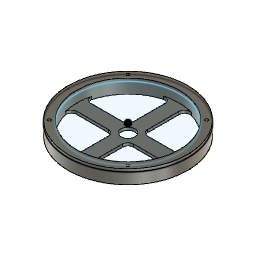
main_body_43mm_diameter v2 (Autodesk Fusion 360 design; units mm, degrees)
Autodesk Fusion 360 part; units mm, degrees
sketch "Sketch1" plane through (0, 0, 0) normal (0, 0, 1) x (1, 0, 0)
  circle A0 centre (0, 0) radius 21.5
  circle A1 centre (0, 0) radius 18.5
  circle A2 centre (0, 0) radius 2.5
  line L0 (-2.5, 4.5) -> (-2.5, 15.8622)
  line L1 (2.5, 15.8622) -> (2.5, 4.5)
  line L2 (4.5, -2.5) -> (15.8806, -2.5)
  line L3 (15.8806, 2.5) -> (4.5, 2.5)
  line L4 (-2.5, -4.5) -> (-2.5, -15.8473)
  line L5 (2.5, -15.8473) -> (2.5, -4.5)
  line L6 (-4.5, -2.5) -> (-15.892, -2.5)
  line L7 (-15.9057, 2.5) -> (-4.5, 2.5)
  arc A3 (2.5, 4.5) -> (4.5, 2.5) centre (4.5, 4.5) ccw
  arc A4 (4.5, -2.5) -> (2.5, -4.5) centre (4.5, -4.5) ccw
  arc A5 (-2.5, -4.5) -> (-4.5, -2.5) centre (-4.5, -4.5) ccw
  arc A6 (-4.5, 2.5) -> (-2.5, 4.5) centre (-4.5, 4.5) ccw
  line L8 (-17.8692, 4.8804) -> (-17.9378, 4.526)
  line L9 (-17.8533, -4.8912) -> (-17.8867, -4.7239)
  arc A7 (-17.8692, 4.8804) -> (-15.9057, 2.5) centre (-15.9057, 4.5) ccw
  arc A8 (-15.892, -2.5) -> (-17.8533, -4.8912) centre (-15.892, -4.5) ccw
  line L10 (-4.926, -17.8014) -> (-5.3564, -17.7076)
  line L11 (4.926, -17.8014) -> (5.3564, -17.7076)
  arc A9 (-4.926, -17.8014) -> (-2.5, -15.8473) centre (-4.5, -15.8473) ccw
  arc A10 (2.5, -15.8473) -> (4.926, -17.8014) centre (4.5, -15.8473) ccw
  line L12 (17.8401, -4.9002) -> (17.8428, -4.8872)
  line L13 (17.8401, 4.9002) -> (17.8428, 4.8872)
  arc A11 (15.8806, 2.5) -> (17.8401, 4.9002) centre (15.8806, 4.5) ccw
  arc A12 (17.8401, -4.9002) -> (15.8806, -2.5) centre (15.8806, -4.5) ccw
  line L14 (4.9145, 17.8188) -> (5.1482, 17.7693)
  line L15 (-4.9145, 17.8188) -> (-5.1482, 17.7693)
  arc A13 (-2.5, 15.8622) -> (-4.9145, 17.8188) centre (-4.5, 15.8622) ccw
  arc A14 (4.9145, 17.8188) -> (2.5, 15.8622) centre (4.5, 15.8622) ccw
  dimension "d1" = 43
  dimension "d2" = 37
  dimension "d3" = 5
  dimension "d6" = 2
  dimension "d7" = 2
  dimension "d8" = 2
  dimension "d9" = 2
  dimension "d10" = 2
  dimension "d11" = 2
  dimension "d12" = 2
  dimension "d13" = 2
  dimension "d14" = 2
  dimension "d15" = 2
  dimension "d16" = 2
  dimension "d17" = 2
  constraint concentric A0 A1
  constraint concentric A1 A2
  constraint vertical L0
  constraint vertical L1
  constraint horizontal L2
  constraint horizontal L3
  constraint vertical L4
  constraint vertical L5
  constraint horizontal L6
  constraint horizontal L7
  constraint tangent L1 A3
  constraint tangent L3 A3
  constraint tangent L2 A4
  constraint tangent L5 A4
  constraint tangent L6 A5
  constraint tangent L4 A5
  constraint tangent L7 A6
  constraint tangent L0 A6
  constraint coincident A1 L8.end
  constraint coincident A1 L9.end
  constraint tangent L8 A7
  constraint tangent L7 A7
  constraint tangent L9 A8
  constraint tangent L6 A8
  constraint coincident A1 L10.end
  constraint coincident A1 L11.end
  constraint tangent L10 A9
  constraint tangent L4 A9
  constraint tangent L11 A10
  constraint tangent L5 A10
  constraint coincident A1 L12.end
  constraint coincident A1 L13.end
  constraint tangent L13 A11
  constraint tangent L3 A11
  constraint tangent L12 A12
  constraint tangent L2 A12
  constraint coincident A1 L14.end
  constraint coincident A1 L15.end
  constraint tangent L15 A13
  constraint tangent L0 A13
  constraint tangent L14 A14
  constraint tangent L1 A14
  measures "d1" diameter of A0
  measures "d2" diameter of A1
  measures "d3" diameter of A2
  measures "d6" radius of A3
  measures "d7" radius of A4
  measures "d8" radius of A5
  measures "d9" radius of A6
  measures "d10" radius of A7
  measures "d11" radius of A8
  measures "d12" radius of A9
  measures "d13" radius of A10
  measures "d14" radius of A11
  measures "d15" radius of A12
  measures "d16" radius of A13
  measures "d17" radius of A14
extrude "Extrude1" add sketch "Sketch1" along normal blind 1 contours A1 L0 L1 L2 L3 L4 L5 L6 L7 A3 A4 A5 A6 A7 A8 L10 L11 A9 A10 A11 A12 L14 L15 A13 A14
sketch "Sketch2" plane through (0, 0, 0) normal (0, 0, 1) x (1, 0, 0)
  circle A0 centre (0, 0) radius 21.5
  circle A1 centre (0, 0) radius 18.5
  line L0 (0, 0) -> (20, 0) construction
  circle A2 centre (-14.1421, 14.1421) radius 0.5
  circle A3 centre (14.1421, 14.1421) radius 0.5
  circle A4 centre (14.1421, -14.1421) radius 0.5
  circle A5 centre (-14.1421, -14.1421) radius 0.5
  dimension "d20" = 43
  dimension "d21" = 37
  dimension "d24" = 1
  dimension "d25" = 1
  dimension "d26" = 1
  dimension "d27" = 1
  constraint coincident A0.centre A1.centre
  constraint concentric A0 A1
  constraint horizontal L0
  measures "d20" diameter of A0
  measures "d21" diameter of A1
  measures "d24" diameter of A2
  measures "d25" diameter of A3
  measures "d26" diameter of A4
  measures "d27" diameter of A5
extrude "Extrude2" add sketch "Sketch2" along normal blind 4
sketch "Sketch3" plane through (0, 0, 4) normal (0, 0, 1) x (-1, 0, 0)
  circle A0 centre (-14.1421, 14.1421) radius 0.5
  circle A1 centre (14.1421, -14.1421) radius 0.5
  circle A2 centre (14.1421, 14.1421) radius 0.5
  circle A3 centre (-14.1421, -14.1421) radius 0.5
  circle A4 centre (0, 0) radius 18.5
  circle A5 centre (0, 0) radius 21.5
sketch "Sketch4" plane through (0, 0, 4) normal (0, 0, 1) x (-1, 0, 0)
  circle A0 centre (0, 0) radius 21.5
  circle A1 centre (0, 0) radius 18.5166
  dimension "d30" = 43
  constraint coincident A0.centre A1.centre
  constraint concentric A0 A1
  measures "d30" diameter of A0
extrude "Extrude3" add sketch "Sketch3" along normal blind 1
